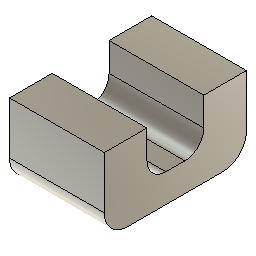
cable holder (Autodesk Fusion 360 design; units mm, degrees)
Autodesk Fusion 360 part; units mm, degrees
sketch "Sketch1" plane through (0, 0, 0) normal (0, 0, 1) x (1, 0, 0)
  line L0 (5, 7.5) -> (-5, 7.5)
  line L1 (-5, 7.5) -> (-5, -7.5)
  line L2 (-5, -7.5) -> (5, -7.5)
  line L3 (5, -7.5) -> (5, 7.5)
  line L4 (5, 7.5) -> (-5, -7.5) construction
  line L5 (-5, 7.5) -> (5, -7.5) construction
  line L6 (-5, 7.5) -> (5, 7.5)
  line L7 (5, 7.5) -> (5, 3)
  line L8 (5, 3) -> (-5, 3)
  line L9 (-5, 3) -> (-5, 7.5)
  line L10 (-5, -7.5) -> (5, -7.5)
  line L11 (5, -7.5) -> (5, -3)
  line L12 (5, -3) -> (-5, -3)
  line L13 (-5, -3) -> (-5, -7.5)
  dimension "d1" = 10
  dimension "d2" = 15
  dimension "d3" = 4.5
  dimension "d4" = 4.5
  constraint horizontal L0
  constraint perpendicular L0 L1
  constraint parallel L0 L2
  constraint parallel L1 L3
  constraint coincident L4 origin
  constraint coincident L5 origin
  constraint horizontal L6
  constraint vertical L7
  constraint horizontal L8
  constraint vertical L9
  constraint coincident L3 L7.end
  constraint horizontal L10
  constraint vertical L11
  constraint horizontal L12
  constraint vertical L13
  measures "d1" distance of L1.end L2.end
  measures "d2" distance of L0.end L1.end
  measures "d3" distance of L0.start L7.end
  measures "d4" distance of L1.end L12.end
extrude "Extrude1" add sketch "Sketch1" along normal blind 3 makes body 1
extrude "Extrude2" add sketch "Sketch1" along normal blind 8 contours L0 L1 L3 L6 L7 L8 L9 | L1 L2 L3 L10 L11 L12 L13 bodies 1
fillet "Fillet1" radius 2 2 edges at (0, -3, 3) (0, 3, 3) on bodies 1
fillet "Fillet2" radius 2.5 2 edges at (0, -7.5, 0) (0, 7.5, 0) on bodies 1
sketch "Sketch2" plane through (0, 0, 0) normal (0, 0, 1) x (1, 0, 0)
  circle A0 centre (20, 0) radius 4
  circle A1 centre (20, 0) radius 9
  dimension "d13" = 8
  dimension "d14" = 18
  constraint concentric A0 A1
  measures "d13" diameter of A0
  measures "d14" diameter of A1
extrude "Extrude3" add sketch "Sketch2" along normal blind 20 separate body makes body 2
delete_body "RemoveBody1" bodies 2
